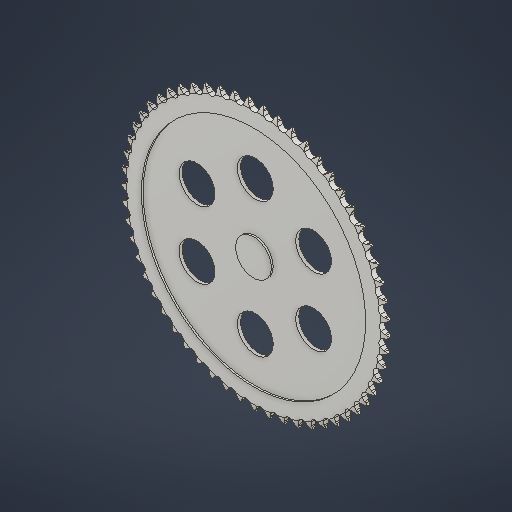
# Autodesk Inventor part: Roller Chain Sprocket2
Saved by Autodesk Inventor 2026.1 (Build 301233020, 233B)
## iProperties
Created: 2025-12-30
Part Number: Roller Chain Sprocket2
Material: Steel
Document SubType Name: Modeling
Designer: Austin Ngobeni
Density: 1 g/cm^3
Appearance: Steel
CustomPartVersion: 1
Author: Austin Ngobeni
Autodesk Inventor part; units mm, degrees
ref_plane "YZ Plane" through (0, 0, 0) normal (1, 0, 0) x (0, 1, 0)
ref_plane "XZ Plane" through (0, 0, 0) normal (0, 1, 0) x (-1, 0, 0)
ref_plane "XY Plane" through (0, 0, 0) normal (0, 0, 1) x (1, 0, 0)
sketch "Theoretical Tooth Profile" plane through (0, 0, 0) normal (0, 0, 1) x (1, 0, 0)
  circle A0 centre (0, 0) radius 72.6114 construction
  line L0 (0, 0) -> (0, 72.6114) construction
  line L1 (0, 0) -> (7.9879, 72.1707) construction
  circle A1 centre (0, 0) radius 74.9012
  arc A2 (-2.0414, 71.1254) -> (2.0414, 71.1254) centre (0, 72.6114) ccw
  line L2 (0, 72.6114) -> (7.9879, 72.1707) construction
  line L3 (0, 72.6114) -> (3.2339, 74.9655) construction
  line L4 (3.2339, 74.9655) -> (-2.9343, 72.8374) construction
  arc A3 (3.8853, 74.8003) -> (3.1771, 73.5411) centre (6.9894, 72.2258) ccw
  arc A4 (-3.1771, 73.5411) -> (-3.8853, 74.8003) centre (-6.9894, 72.2258) ccw
  line L5 (-6.9894, 72.2258) -> (-3.1771, 73.5411) construction
  arc A5 (-2.9343, 72.8374) -> (-2.0414, 71.1254) centre (3.2339, 74.9655) ccw
  line L6 (-2.9343, 72.8374) -> (-3.1771, 73.5411)
  arc A6 (2.0414, 71.1254) -> (2.9343, 72.8374) centre (-3.2339, 74.9655) ccw
  line L7 (3.1771, 73.5411) -> (2.9343, 72.8374)
  line L8 (0, 0) -> (4.1261, 74.7874) construction
  point P0 (3.9939, 72.3911)
  dimension "d0" = 145.2228
  dimension "d2" = 6.316
  dimension "d3" = 2.525
  dimension "d10" = 126.053
  dimension "d11" = 17.017
  dimension "d12" = 4
  dimension "d13" = 6.525
  dimension "d14" = 7
  dimension "d23" = 2.4
  constraints: 18 end point, 15 point on circle, 7 centre point, 3 coincident, 3 point on line, 3 symmetric about line, 3 tangent, 1 equal radius, 1 midpoint, 1 parallel, 1 vertical, 1 other
  measures "d0" diameter of A0
  measures "d2" angle of L1 L0
  measures "d3" radius of A2
  measures "d10" angle of L3 L0
  measures "d11" angle of L4 L3
  measures "d12" distance of L2.start L3.end
  measures "d13" distance of L3.end L4.end
  measures "d14" distance of A3.centre L0.end
  measures "d23" distance from line of L8.end L2
sketch "Tooth Profile" plane through (0, 0, 0) normal (0, 0, 1) x (1, 0, 0)
  arc A0 (-2.3606, 71.7152) -> (2.3606, 71.7152) centre (0, 72.6114) ccw
  arc A1 (3.7073, 74.8093) -> (2.3606, 71.7152) centre (35.4557, 59.1505) ccw
  arc A2 (-2.3606, 71.7152) -> (-3.7073, 74.8093) centre (-35.4557, 59.1505) ccw
  line L0 (0, 0) -> (0, 72.6114) construction
  line L1 (0, 72.6114) -> (2.3606, 71.7152) construction
  line L2 (0, 72.6114) -> (-2.3606, 71.7152) construction
  circle A3 centre (0, 0) radius 74.9012 projected
  dimension "d44" = 138.421
  dimension "d45" = 35.4
  dimension "d46" = 2.525
  constraints: 9 point on circle, 6 end point, 3 centre point, 2 tangent, 1 coincident, 1 equal radius, 1 vertical, 1 other
  measures "d44" angle of L2 L1
  measures "d45" radius of A1
  measures "d46" radius of A0
sketch "Section Profile" plane through (0, 0, 0) normal (1, 0, 0) x (0, 1, 0)
  line L0 (74.9012, 0) -> (-74.9012, 0) projected
  line L1 (64.684, 1.395) -> (-64.684, 1.395)
  line L2 (-64.684, 1.395) -> (-64.684, -1.395)
  line L3 (-64.684, -1.395) -> (64.684, -1.395)
  line L4 (64.684, -1.395) -> (64.684, 1.395)
  line L5 (64.684, 1.395) -> (74.9012, 1.395) construction
  line L6 (74.9012, 1.395) -> (74.9012, -1.395) construction
  line L7 (74.9012, -1.395) -> (64.684, -1.395) construction
  line L8 (64.684, -1.395) -> (64.684, 1.395)
  arc A0 (74.9012, 0.355) -> (70.9567, 1.395) centre (70.9567, -6.605) ccw
  arc A1 (70.9567, -1.395) -> (74.9012, -0.355) centre (70.9567, 6.605) ccw
  line L9 (70.9567, 1.395) -> (0, 1.395)
  line L10 (0, 1.395) -> (0, -1.395)
  line L11 (0, -1.395) -> (70.9567, -1.395)
  line L12 (0, 1.395) -> (0, -1.395)
  line L13 (74.9012, 0.355) -> (74.9012, -0.355)
  point P0 (0, 0)
  point P1 (0, 0)
  dimension "d30" = 2.79
  dimension "d31" = 129.3679
  dimension "d32" = 2.79
  dimension "d33" = 1.04
  dimension "d34" = 8
  dimension "d43" = 1.395
  constraints: 26 end point, 7 midpoint, 5 perpendicular, 4 parallel, 4 point on circle, 3 point on line, 3 symmetric about line, 2 centre point, 2 horizontal, 2 tangent, 1 collinear, 1 other
  measures "d30" distance between parallel lines of L7 L5
  measures "d31" distance between parallel lines of L2 L4
  measures "d32" distance between parallel lines of L3 L1
  measures "d33" distance from line of L13.start L5
  measures "d34" radius of A0
  measures "d43" distance between parallel lines of L3 L0
revolve "Shroud" add sketch "Section Profile" angle 360 about axis through (0, 0, 1.395) along (0, 0, -1) contours L10 L3 L2 L0 | L0 L2 L1 L10
revolve "Strand" add sketch "Section Profile" angle 360 about axis through (0, 0, 1.395) along (0, 0, -1) contours L13 A1 L11 L4 L0 | L0 L4 L9 A0 L13 | L4 L3 L10 L0 | L0 L10 L1 L4
fillet "Fillet2" [suppressed]
pattern_of_one "Strand Pattern"
extrude "Theoretical Tooth" cut sketch "Theoretical Tooth Profile" along normal through all both and the other way through all contours A3 L7 A6 A2 A5 L6 A4 A1 picked at (0.4319, 72.3803)
extrude "Tooth" [suppressed]
pattern_circular "Tooth Pattern" count 57 over 360 about axis through (0, 0, -10) along (0, 0, 1) of "Theoretical Tooth"
ref_plane "Timing Plane" through (0, 72.6114, 0) normal (1, 0, 0) x (0, 1, 0)
sketch "Sketch4" plane through (0, 72.6114, 1.395) normal (0, 0, 1) x (1, 0, 0)
  circle A0 centre (0, -72.6114) radius 62.5
  circle A1 centre (0, -72.6114) radius 10
  circle A2 centre (0, -72.6114) radius 37.5 construction
  circle A3 centre (0, -35.1114) radius 10
  circle A4 centre (0, -72.6114) radius 37.5 construction
  circle A5 centre (-32.476, -53.8614) radius 10
  circle A6 centre (0, -72.6114) radius 37.5 construction
  circle A7 centre (-32.476, -91.3614) radius 10
  circle A8 centre (0, -72.6114) radius 37.5 construction
  circle A9 centre (0, -110.1114) radius 10
  circle A10 centre (0, -72.6114) radius 37.5 construction
  circle A11 centre (32.476, -91.3614) radius 10
  circle A12 centre (0, -72.6114) radius 37.5 construction
  circle A13 centre (32.476, -53.8614) radius 10
  dimension "d55" = 75
  dimension "d53" = 125
  dimension "d54" = 20
  dimension "d56" = 20
  dimension "d59" = 360
  constraints: 8 centre point, 3 coincident, 2 vertical alignment, 41 other
  measures "d53" diameter of A0
  measures "d54" diameter of A1
  measures "d56" diameter of A3
extrude "Extrusion4" cut sketch "Sketch4" against normal blind 1
extrude "Extrusion5" cut sketch "Sketch4" against normal through all contours A3 | A5 | A7 | A9 | A11 | A13
equation "\"d3\" = 0.5 * da_Dr + da_SC"
equation "\"d12\" = 0.8 * da_Dr"
equation "\"d13\" = 1.3 * da_Dr + da_SC"
equation "\"d14\" = 1.4 * da_Dr"
equation "\"d23\" = da_Ha"
equation "\"d44\" = da_Alfa"
equation "\"d45\" = da_Re"
equation "\"d46\" = da_Ri"
equation "\"d30\" = da_Bf"
equation "\"d31\" = da_Ds"
equation "\"d32\" = da_Bs"
equation "\"d33\" = da_Ba"
equation "\"d34\" = da_Rx"
equation "\"d51\" = da_Ra"
equation "\"d40\" = da_pt"
equation "\"form_type\" = 0"
equation "\"da_p\" = 8"
equation "\"da_Dr\" = 5"
equation "\"da_SC\" = 0.025"
equation "\"da_Ha\" = 2.4"
equation "\"da_pt\" = 5.64"
equation "\"da_Bf\" = 2.79"
equation "\"da_Ba\" = 1.04"
equation "\"da_Rx\" = 8"
equation "\"da_Ra\" = 0.32"
equation "\"da_Bs\" = 2.79"
equation "\"da_Ds\" = 129.3679"
equation "\"da_Re\" = 35.4"
equation "\"da_Ri\" = 2.525"
equation "\"da_Alfa\" = 138.421deg"
body "Solid1"
